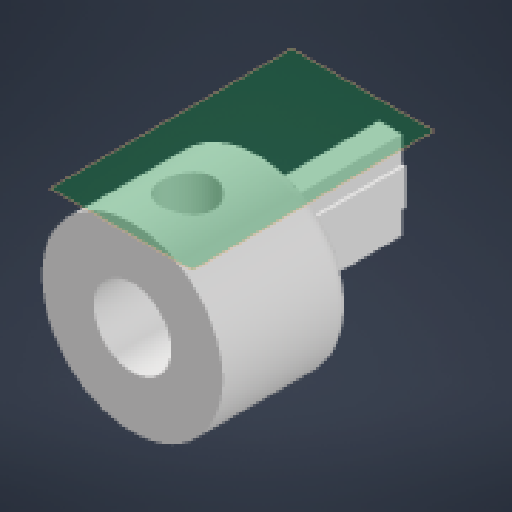
# Autodesk Inventor part: Pot_adapter
Saved by Autodesk Inventor 2026.1 (Build 301233020, 233B)
## iProperties
Created: 2025-11-11
Part Number: Pot_adapter
Material: Generic
Document SubType Name: Modeling
Designer: Mikke
Density: 1 g/cm^3
Appearance: Default
Author: Mikke
Autodesk Inventor part; units mm, degrees
ref_plane "YZ Plane" through (0, 0, 0) normal (1, 0, 0) x (0, 1, 0)
ref_plane "XZ Plane" through (0, 0, 0) normal (0, 1, 0) x (-1, 0, 0)
ref_plane "XY Plane" through (0, 0, 0) normal (0, 0, 1) x (1, 0, 0)
sketch "Sketch1" plane through (0, 0, 0) normal (0, 0, 1) x (1, 0, 0)
  line L0 (1.25, -1.5) -> (1, -1.5) projected
  line L1 (1, -1.5) -> (1, -3.5) projected
  line L2 (1, -3.5) -> (-1, -3.5) projected
  line L3 (-1, -3.5) -> (-1, -1.5) projected
  line L4 (-1, -1.5) -> (-1.25, -1.5) projected
  line L5 (-1.25, -1.5) -> (-1.25, 1.5) projected
  line L6 (-1.25, 1.5) -> (-1, 1.5) projected
  line L7 (-1, 1.5) -> (-1, 3.5) projected
  line L8 (-1, 3.5) -> (1, 3.5) projected
  line L9 (1, 3.5) -> (1, 1.5) projected
  line L10 (1, 1.5) -> (1.25, 1.5) projected
  line L11 (1.25, 1.5) -> (1.25, -1.5) projected
  circle A0 centre (4.5, 0) radius 1.55 projected
  circle A1 centre (-4.5, 0) radius 1.55 projected
  circle A2 centre (0, 0) radius 8 projected
  line L12 (-0.9, -1.4) -> (-0.9, -3.4)
  line L13 (-0.9, -3.4) -> (0.9, -3.4)
  line L14 (0.9, -3.4) -> (0.9, -1.4)
  line L15 (0.9, -1.4) -> (1.15, -1.4)
  line L16 (1.15, -1.4) -> (1.15, 1.4)
  line L17 (1.15, 1.4) -> (0.9, 1.4)
  line L18 (0.9, 1.4) -> (0.9, 3.4)
  line L19 (0.9, 3.4) -> (-0.9, 3.4)
  line L20 (-0.9, 3.4) -> (-0.9, 1.4)
  line L21 (-0.9, 1.4) -> (-1.15, 1.4)
  line L22 (-1.15, 1.4) -> (-1.15, -1.4)
  line L23 (-1.15, -1.4) -> (-0.9, -1.4)
  point P0 (0, 0)
  dimension "d0" = 0.1
  constraints: 24 end point, 11 other
  measures "d0" distance between parallel lines of L3 L12
extrude "Extrusion1" add sketch "Sketch1" against normal blind 7 contours L23 L22 L21 L20 L19 L18 L17 L16 L15 L14 L13 L12
sketch "Sketch2" plane through (0, 0, 0) normal (0, 0, 1) x (1, 0, 0)
  line L0 (-0.9, -3.4) -> (0.9, -3.4) projected
  line L1 (0.9, -3.4) -> (0.9, -1.4) projected
  line L2 (0.9, -1.4) -> (1.15, -1.4) projected
  line L3 (1.15, -1.4) -> (1.15, 1.4) projected
  line L4 (1.15, 1.4) -> (0.9, 1.4) projected
  line L5 (0.9, 1.4) -> (0.9, 3.4) projected
  line L6 (0.9, 3.4) -> (-0.9, 3.4) projected
  line L7 (-0.9, 3.4) -> (-0.9, 1.4) projected
  line L8 (-0.9, 1.4) -> (-1.15, 1.4) projected
  line L9 (-1.15, 1.4) -> (-1.15, -1.4) projected
  line L10 (-1.15, -1.4) -> (-0.9, -1.4) projected
  line L11 (-0.9, -1.4) -> (-0.9, -3.4) projected
  point P0 (0, 0)
extrude "Extrusion2" add sketch "Sketch2" along normal blind 3
sketch "Sketch3" plane through (0, 0, 3) normal (0, 0, 1) x (1, 0, 0)
  circle A0 centre (0, 0) radius 3
  line L0 (0, 0) -> (-1.5, 0)
  line L1 (-1.5, -2.5981) -> (-1.5, 2.5981)
  line L2 (-1.5, -2.5981) -> (3.6962, -2.5981) construction
  circle A1 centre (0, 0) radius 7
  dimension "d5" = 6
  dimension "d6" = 1.5
  dimension "d7" = 90
  dimension "d8" = 14
  constraints: 6 end point, 2 coincident, 2 horizontal, 1 centre point, 1 midpoint, 1 perpendicular, 3 other
  measures "d6" distance of L0.start L0.end
  measures "d7" angle of L2 L1
  measures "d8" diameter of A1
extrude "Extrusion3" add sketch "Sketch3" along normal blind 2 contours A0 L1 | L1 A0 | A1
sketch "Sketch4" plane through (0, 0, 5) normal (0, 0, 1) x (1, 0, 0)
  circle A0 centre (0, 0) radius 3
  line L0 (0, 0) -> (0, -1.5)
  line L1 (2.5981, -1.5) -> (-2.5981, -1.5)
  circle A1 centre (0, 0) radius 7 projected
  dimension "d11" = 6
  dimension "d12" = 1.5
  constraints: 4 end point, 1 coincident, 1 horizontal, 1 midpoint, 1 vertical, 3 other
  measures "d12" distance of L0.start L0.end
extrude "Extrusion4" add sketch "Sketch4" along normal blind 10
fillet "Fillet1" radius 1 1 edges at (-7, 0, 3)
fillet "Fillet2" radius 1 4 edges at (0, -3.4, 3) (1.15, 0, 3) (-1.15, 0, 3) (0, 3.4, 3)
sketch "Sketch6" plane through (0, 0, 15) normal (0, 0, 1) x (1, 0, 0)
  circle A0 centre (0, 0) radius 5 projected
  circle A1 centre (0, 0) radius 3 projected
  circle A2 centre (0, 0) radius 3 projected
  circle A3 centre (0, 0) radius 7
  point P0 (-2.5981, -1.5)
  point P1 (2.5981, -1.5)
  constraints: 1 centre point, 1 coincident
extrude "Extrusion6" cut sketch "Sketch6" against normal blind 2 contours A0 | A1 | A3
ref_plane "Work Plane2" through (0, 7, 3) normal (0, -1, 0) x (1, 0, 0)
ref_plane "Work Plane1" through (20.4658, -7.5, 10.75) normal (0, -1, 0) x (1, 0, 0)
sketch "Sketch8" plane through (0, 7, 3) normal (0, -1, 0) x (1, 0, 0)
  circle A0 centre (0, 5.7603) radius 2
  point P0 (0, -3)
  dimension "d22" = 4
  constraints: 1 centre point
  measures "d22" diameter of A0
extrude "Extrusion7" cut sketch "Sketch8" along normal blind 5
body "Solid1"
